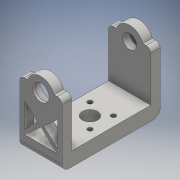
# Autodesk Inventor part: ServoArm
Saved by Autodesk Inventor 2016 (Build 200138000, 138)
## iProperties
Created: 2016-11-10
Part Number: ServoArm
Material: 一般
Document SubType Name: Modeling
Designer: Daisuke
Density: 1 g/cm^3
Appearance: 既定
Author: Daisuke
Autodesk Inventor part; units mm, degrees
ref_plane "YZ Plane" through (0, 0, 0) normal (1, 0, 0) x (0, 1, 0)
ref_plane "XZ Plane" through (0, 0, 0) normal (0, 1, 0) x (-1, 0, 0)
ref_plane "XY Plane" through (0, 0, 0) normal (0, 0, 1) x (1, 0, 0)
sketch "スケッチ1" plane through (0, 0, 0) normal (0, 0, 1) x (1, 0, 0)
  line L0 (-9, 20.9) -> (9, 20.9)
  line L1 (9, 20.9) -> (9, -20.9)
  line L2 (9, -20.9) -> (-9, -20.9)
  line L3 (-9, -20.9) -> (-9, 20.9)
  line L4 (-9, 20.9) -> (9, -20.9) construction
  line L5 (9, 20.9) -> (-9, -20.9) construction
  circle A0 centre (0, 0) radius 3.25
  line L6 (-5, 5) -> (5, 5) construction
  line L7 (5, 5) -> (5, -5) construction
  line L8 (5, -5) -> (-5, -5) construction
  line L9 (-5, -5) -> (-5, 5) construction
  line L10 (-5, 5) -> (5, -5) construction
  line L11 (5, 5) -> (-5, -5) construction
  circle A1 centre (5, 5) radius 1
  circle A2 centre (-5, 5) radius 1
  circle A3 centre (-5, -5) radius 1
  circle A4 centre (5, -5) radius 1
  dimension "d0" = 18
  dimension "d1" = 41.8
  dimension "d2" = 6.5
  dimension "d3" = 10
  dimension "d4" = 10
  dimension "d5" = 2
  dimension "d6" = 2
  dimension "d7" = 2
  dimension "d8" = 2
  constraints: 24 end point, 5 centre point, 5 coincident, 4 midpoint, 4 parallel, 2 horizontal, 2 perpendicular
  measures "d0" distance of L1.end L2.end
  measures "d1" distance of L0.end L1.end
  measures "d2" diameter of A0
  measures "d3" distance of L7.end L8.end
  measures "d4" distance of L6.end L7.end
  measures "d5" diameter of A1
  measures "d6" diameter of A2
  measures "d7" diameter of A3
  measures "d8" diameter of A4
extrude "押し出し1" add sketch "スケッチ1" along normal blind 6
sketch "スケッチ2" plane through (0, 0, 6) normal (0, 0, 1) x (1, 0, 0)
  line L0 (-9, 20.9) -> (9, 20.9)
  line L1 (-9, 9) -> (-9, 20.9)
  line L2 (9, 20.9) -> (-9, 20.9)
  line L3 (-9, 20.9) -> (-9, 16.9)
  line L4 (-9, 16.9) -> (9, 16.9)
  line L5 (9, 16.9) -> (9, 20.9)
  line L6 (9, -9) -> (9, -20.9)
  line L7 (-9, -20.9) -> (-9, -9)
  line L8 (9, -20.9) -> (-9, -20.9)
  line L9 (-9, -20.9) -> (-9, -16.9)
  line L10 (-9, -16.9) -> (9, -16.9)
  line L11 (9, -16.9) -> (9, -20.9)
  point P0 (0, 0)
  point P1 (0, 0)
  dimension "d11" = 4
  dimension "d12" = 4
  constraints: 24 end point, 4 parallel, 2 horizontal, 2 perpendicular, 2 point on line
  measures "d11" distance of L3.end L2.end
  measures "d12" distance of L8.end L9.end
extrude "押し出し2" add sketch "スケッチ2" along normal blind 25
sketch "スケッチ3" plane through (-9, 20.9, 0) normal (0, 1, 0) x (1, 0, 0)
  line L0 (18, -31) -> (18, 0)
  line L1 (0, 0) -> (18, 0)
  line L2 (18, 0) -> (0, 0)
  line L3 (18, -31) -> (18, -25) construction
  line L4 (18, -25) -> (18, -31)
  line L5 (9, -25) -> (15, -25) construction
  line L6 (9, -25) -> (18, -25) construction
  line L7 (16, -27) -> (18, -27)
  line L8 (14.6569, -27) -> (16, -27)
  line L9 (9, -25) -> (9, -31) construction
  line L10 (2, -27) -> (3.3431, -27)
  line L11 (9, -25) -> (0, -25) construction
  line L12 (0, -25) -> (0, -31) construction
  line L13 (0, -25) -> (0, -31)
  circle A0 centre (9, -25) radius 6
  line L14 (18, -6) -> (18, -31)
  line L15 (0, -6) -> (0, -31) construction
  line L16 (18, 0) -> (18, -31) construction
  line L17 (9, 0) -> (9, -25) construction
  line L18 (0, 0) -> (0, -31)
  line L19 (0, -6) -> (0, -31) construction
  line L20 (18, -31) -> (0, -31) construction
  line L21 (0, -31) -> (18, -31) construction
  line L22 (0, -31) -> (18, -31)
  line L23 (18, -31) -> (0, -31) construction
  line L24 (0, -31) -> (18, -31) construction
  line L25 (0, -25) -> (2, -25) construction
  line L26 (2, -25) -> (0, -25) construction
  line L27 (18, -25) -> (16, -25) construction
  line L28 (2, -27) -> (0, -27)
  line L29 (18, -31) -> (18, 0)
  line L30 (0, 0) -> (18, 0)
  line L31 (18, 0) -> (0, 0)
  line L32 (18, -31) -> (18, -25) construction
  line L33 (18, -25) -> (18, -31)
  line L34 (9, -25) -> (15, -25) construction
  line L35 (9, -25) -> (18, -25) construction
  line L36 (16, -27) -> (18, -27)
  line L37 (14.6569, -27) -> (16, -27)
  line L38 (9, -25) -> (9, -31) construction
  line L39 (2, -27) -> (3.3431, -27)
  line L40 (9, -25) -> (0, -25) construction
  line L41 (0, -25) -> (0, -31) construction
  line L42 (0, -25) -> (0, -31)
  circle A1 centre (9, -25) radius 6
  line L43 (18, -6) -> (18, -31)
  line L44 (0, -6) -> (0, -31) construction
  line L45 (18, 0) -> (18, -31) construction
  line L46 (9, 0) -> (9, -25) construction
  line L47 (0, 0) -> (0, -31)
  line L48 (0, -6) -> (0, -31) construction
  line L49 (18, -31) -> (0, -31) construction
  line L50 (0, -31) -> (18, -31) construction
  line L51 (0, -31) -> (18, -31)
  line L52 (18, -31) -> (0, -31) construction
  line L53 (0, -31) -> (18, -31) construction
  line L54 (0, -25) -> (2, -25) construction
  line L55 (2, -25) -> (0, -25) construction
  line L56 (18, -25) -> (16, -25) construction
  line L57 (2, -27) -> (0, -27)
  point P0 (9, -6)
  point P1 (9, -6)
  constraints: 116 end point, 14 point on line, 6 coincident, 4 point on circle, 2 centre point, 2 collinear
extrude "押し出し3" cut sketch "スケッチ3" against normal blind 42 contours L22 A0 L8 L7 L0 | L22 L13 L28 L10 A0
sketch "スケッチ4" plane through (-9, 16.9, 6) normal (0, -1, 0) x (1, 0, 0)
  line L0 (0, 25.0086) -> (0, 19.0086)
  line L1 (0, 25.0086) -> (0, 19.0086) construction
  line L2 (0, 19.0086) -> (0, 25.0086)
  line L3 (9, 19.0086) -> (3, 19.0086) construction
  line L4 (9, 19.0086) -> (0, 19.0086) construction
  line L5 (2, 21.0086) -> (0, 21.0086)
  line L6 (3.3431, 21.0086) -> (2, 21.0086)
  line L7 (9, 19.0086) -> (9, 25.0086) construction
  line L8 (16, 21.0086) -> (14.6569, 21.0086)
  line L9 (9, 19.0086) -> (18, 19.0086) construction
  line L10 (18, 19.0086) -> (18, 25.0086) construction
  line L11 (18, 19.0086) -> (18, 25.0086)
  circle A0 centre (9, 19.0086) radius 6
  line L12 (0, 19.0086) -> (0, 25.0086)
  line L13 (18, 19.0086) -> (18, 25.0086) construction
  line L14 (0, 19.0086) -> (0, 25.0086) construction
  line L15 (9, 0) -> (9, 25) construction
  line L16 (18, 19.0086) -> (18, 25.0086)
  line L17 (18, 0.0086) -> (18, 25.0086) construction
  line L18 (0, 25.0086) -> (18, 25.0086) construction
  line L19 (18, 25.0086) -> (0, 25.0086) construction
  line L20 (18, 25.0086) -> (0, 25.0086)
  line L21 (0, 25.0086) -> (18, 25.0086) construction
  line L22 (18, 25.0086) -> (0, 25.0086) construction
  line L23 (18, 19.0086) -> (16, 19.0086) construction
  line L24 (16, 19.0086) -> (18, 19.0086) construction
  line L25 (0, 19.0086) -> (2, 19.0086) construction
  line L26 (16, 21.0086) -> (18, 21.0086)
  circle A1 centre (9, 19.0086) radius 1.5
  circle A2 centre (9, 19.0086) radius 3
  point P0 (9, -6)
  point P1 (9, 0.0086)
  dimension "d17" = 3
  dimension "d18" = 6
  constraints: 54 end point, 6 point on line, 5 coincident, 3 centre point, 2 point on circle
  measures "d17" diameter of A1
  measures "d18" diameter of A2
extrude "押し出し4" cut sketch "スケッチ4" against normal blind 3 contours A2
sketch "スケッチ5" plane through (-9, 16.9, 6) normal (0, -1, 0) x (1, 0, 0)
  line L0 (0, 25.0086) -> (0, 19.0086)
  line L1 (0, 25.0086) -> (0, 19.0086) construction
  line L2 (0, 19.0086) -> (0, 25.0086)
  line L3 (9, 19.0086) -> (3, 19.0086) construction
  line L4 (9, 19.0086) -> (0, 19.0086) construction
  line L5 (2, 21.0086) -> (0, 21.0086)
  line L6 (3.3431, 21.0086) -> (2, 21.0086)
  line L7 (9, 19.0086) -> (9, 25.0086) construction
  line L8 (16, 21.0086) -> (14.6569, 21.0086)
  line L9 (9, 19.0086) -> (18, 19.0086) construction
  line L10 (18, 19.0086) -> (18, 25.0086) construction
  line L11 (18, 19.0086) -> (18, 25.0086)
  circle A0 centre (9, 19.0086) radius 6
  line L12 (0, 19.0086) -> (0, 25.0086)
  line L13 (18, 19.0086) -> (18, 25.0086) construction
  line L14 (0, 19.0086) -> (0, 25.0086) construction
  line L15 (9, 0) -> (9, 25) construction
  line L16 (18, 19.0086) -> (18, 25.0086)
  line L17 (18, 0.0086) -> (18, 25.0086) construction
  line L18 (0, 25.0086) -> (18, 25.0086) construction
  line L19 (18, 25.0086) -> (0, 25.0086) construction
  line L20 (18, 25.0086) -> (0, 25.0086)
  line L21 (0, 25.0086) -> (18, 25.0086) construction
  line L22 (18, 25.0086) -> (0, 25.0086) construction
  line L23 (18, 19.0086) -> (16, 19.0086) construction
  line L24 (16, 19.0086) -> (18, 19.0086) construction
  line L25 (0, 19.0086) -> (2, 19.0086) construction
  line L26 (16, 21.0086) -> (18, 21.0086)
  circle A1 centre (9, 19.0086) radius 1.5
  circle A2 centre (9, 19.0086) radius 3
  point P0 (9, -6)
  point P1 (9, -6)
  point P2 (9, 0.0086)
  dimension "d21" = 3
  dimension "d22" = 6
  constraints: 54 end point, 6 point on line, 5 coincident, 3 centre point, 2 point on circle
  measures "d21" diameter of A1
  measures "d22" diameter of A2
extrude "押し出し5" cut sketch "スケッチ5" against normal blind 4 contours A1
sketch "スケッチ6" plane through (-9, -16.9, 6) normal (0, 1, 0) x (1, 0, 0)
  line L0 (18, -25.0086) -> (18, -19.0086)
  line L1 (18, -25.0086) -> (18, -19.0086) construction
  line L2 (18, -19.0086) -> (18, -25.0086)
  line L3 (9, -19.0086) -> (15, -19.0086) construction
  line L4 (9, -19.0086) -> (18, -19.0086) construction
  line L5 (16, -21.0086) -> (18, -21.0086)
  line L6 (14.6569, -21.0086) -> (16, -21.0086)
  line L7 (9, -19.0086) -> (9, -25.0086) construction
  line L8 (2, -21.0086) -> (3.3431, -21.0086)
  line L9 (9, -19.0086) -> (0, -19.0086) construction
  line L10 (0, -19.0086) -> (0, -25.0086) construction
  line L11 (0, -19.0086) -> (0, -25.0086)
  circle A0 centre (9, -19.0086) radius 6
  line L12 (18, -19.0086) -> (18, -25.0086)
  line L13 (0, -19.0086) -> (0, -25.0086) construction
  line L14 (18, -19.0086) -> (18, -25.0086) construction
  line L15 (9, 0) -> (9, -25) construction
  line L16 (0, -19.0086) -> (0, -25.0086)
  line L17 (0, -0.0086) -> (0, -25.0086) construction
  line L18 (18, -25.0086) -> (0, -25.0086) construction
  line L19 (0, -25.0086) -> (18, -25.0086) construction
  line L20 (0, -25.0086) -> (18, -25.0086)
  line L21 (18, -25.0086) -> (0, -25.0086) construction
  line L22 (0, -25.0086) -> (18, -25.0086) construction
  line L23 (0, -19.0086) -> (2, -19.0086) construction
  line L24 (2, -19.0086) -> (0, -19.0086) construction
  line L25 (18, -19.0086) -> (16, -19.0086) construction
  line L26 (2, -21.0086) -> (0, -21.0086)
  circle A1 centre (9, -19.0086) radius 3.5
  circle A2 centre (9, -19.0086) radius 4.5
  line L27 (18, -25.0086) -> (18, -19.0086)
  line L28 (18, -25.0086) -> (18, -19.0086) construction
  line L29 (18, -19.0086) -> (18, -25.0086)
  line L30 (9, -19.0086) -> (15, -19.0086) construction
  line L31 (9, -19.0086) -> (18, -19.0086) construction
  line L32 (16, -21.0086) -> (18, -21.0086)
  line L33 (14.6569, -21.0086) -> (16, -21.0086)
  line L34 (9, -19.0086) -> (9, -25.0086) construction
  line L35 (2, -21.0086) -> (3.3431, -21.0086)
  line L36 (9, -19.0086) -> (0, -19.0086) construction
  line L37 (0, -19.0086) -> (0, -25.0086) construction
  line L38 (0, -19.0086) -> (0, -25.0086)
  circle A3 centre (9, -19.0086) radius 6
  line L39 (18, -19.0086) -> (18, -25.0086)
  line L40 (0, -19.0086) -> (0, -25.0086) construction
  line L41 (18, -19.0086) -> (18, -25.0086) construction
  line L42 (9, 0) -> (9, -25) construction
  line L43 (0, -19.0086) -> (0, -25.0086)
  line L44 (0, -0.0086) -> (0, -25.0086) construction
  line L45 (18, -25.0086) -> (0, -25.0086) construction
  line L46 (0, -25.0086) -> (18, -25.0086) construction
  line L47 (0, -25.0086) -> (18, -25.0086)
  line L48 (18, -25.0086) -> (0, -25.0086) construction
  line L49 (0, -25.0086) -> (18, -25.0086) construction
  line L50 (0, -19.0086) -> (2, -19.0086) construction
  line L51 (2, -19.0086) -> (0, -19.0086) construction
  line L52 (18, -19.0086) -> (16, -19.0086) construction
  line L53 (2, -21.0086) -> (0, -21.0086)
  circle A4 centre (9, -19.0086) radius 3.5
  circle A5 centre (9, -19.0086) radius 4.5
  point P0 (9, 6)
  point P1 (9, -0.0086)
  point P2 (9, -0.0086)
  dimension "d25" = 7
  dimension "d26" = 9
  dimension "d27" = 7
  dimension "d28" = 9
  constraints: 108 end point, 12 point on line, 10 coincident, 6 centre point, 4 point on circle
  measures "d25" diameter of A1
  measures "d26" diameter of A2
  measures "d27" diameter of A4
  measures "d28" diameter of A5
extrude "押し出し6" cut sketch "スケッチ6" against normal blind 3 contours A2
sketch "スケッチ7" plane through (-9, -16.9, 6) normal (0, 1, 0) x (1, 0, 0)
  line L0 (18, -25.0086) -> (18, -19.0086)
  line L1 (18, -25.0086) -> (18, -19.0086) construction
  line L2 (18, -19.0086) -> (18, -25.0086)
  line L3 (9, -19.0086) -> (15, -19.0086) construction
  line L4 (9, -19.0086) -> (18, -19.0086) construction
  line L5 (16, -21.0086) -> (18, -21.0086)
  line L6 (14.6569, -21.0086) -> (16, -21.0086)
  line L7 (9, -19.0086) -> (9, -25.0086) construction
  line L8 (2, -21.0086) -> (3.3431, -21.0086)
  line L9 (9, -19.0086) -> (0, -19.0086) construction
  line L10 (0, -19.0086) -> (0, -25.0086) construction
  line L11 (0, -19.0086) -> (0, -25.0086)
  circle A0 centre (9, -19.0086) radius 6
  line L12 (18, -19.0086) -> (18, -25.0086)
  line L13 (0, -19.0086) -> (0, -25.0086) construction
  line L14 (18, -19.0086) -> (18, -25.0086) construction
  line L15 (9, 0) -> (9, -25) construction
  line L16 (0, -19.0086) -> (0, -25.0086)
  line L17 (0, -0.0086) -> (0, -25.0086) construction
  line L18 (18, -25.0086) -> (0, -25.0086) construction
  line L19 (0, -25.0086) -> (18, -25.0086) construction
  line L20 (0, -25.0086) -> (18, -25.0086)
  line L21 (18, -25.0086) -> (0, -25.0086) construction
  line L22 (0, -25.0086) -> (18, -25.0086) construction
  line L23 (0, -19.0086) -> (2, -19.0086) construction
  line L24 (2, -19.0086) -> (0, -19.0086) construction
  line L25 (18, -19.0086) -> (16, -19.0086) construction
  line L26 (2, -21.0086) -> (0, -21.0086)
  circle A1 centre (9, -19.0086) radius 3.5
  circle A2 centre (9, -19.0086) radius 4.5
  line L27 (18, -25.0086) -> (18, -19.0086)
  line L28 (18, -25.0086) -> (18, -19.0086) construction
  line L29 (18, -19.0086) -> (18, -25.0086)
  line L30 (9, -19.0086) -> (15, -19.0086) construction
  line L31 (9, -19.0086) -> (18, -19.0086) construction
  line L32 (16, -21.0086) -> (18, -21.0086)
  line L33 (14.6569, -21.0086) -> (16, -21.0086)
  line L34 (9, -19.0086) -> (9, -25.0086) construction
  line L35 (2, -21.0086) -> (3.3431, -21.0086)
  line L36 (9, -19.0086) -> (0, -19.0086) construction
  line L37 (0, -19.0086) -> (0, -25.0086) construction
  line L38 (0, -19.0086) -> (0, -25.0086)
  circle A3 centre (9, -19.0086) radius 6
  line L39 (18, -19.0086) -> (18, -25.0086)
  line L40 (0, -19.0086) -> (0, -25.0086) construction
  line L41 (18, -19.0086) -> (18, -25.0086) construction
  line L42 (9, 0) -> (9, -25) construction
  line L43 (0, -19.0086) -> (0, -25.0086)
  line L44 (0, -0.0086) -> (0, -25.0086) construction
  line L45 (18, -25.0086) -> (0, -25.0086) construction
  line L46 (0, -25.0086) -> (18, -25.0086) construction
  line L47 (0, -25.0086) -> (18, -25.0086)
  line L48 (18, -25.0086) -> (0, -25.0086) construction
  line L49 (0, -25.0086) -> (18, -25.0086) construction
  line L50 (0, -19.0086) -> (2, -19.0086) construction
  line L51 (2, -19.0086) -> (0, -19.0086) construction
  line L52 (18, -19.0086) -> (16, -19.0086) construction
  line L53 (2, -21.0086) -> (0, -21.0086)
  circle A4 centre (9, -19.0086) radius 3.5
  circle A5 centre (9, -19.0086) radius 4.5
  point P0 (9, 6)
  point P1 (9, 6)
  point P2 (9, -0.0086)
  point P3 (9, -0.0086)
  dimension "d31" = 7
  dimension "d32" = 9
  dimension "d33" = 7
  dimension "d34" = 9
  constraints: 108 end point, 12 point on line, 10 coincident, 6 centre point, 4 point on circle
  measures "d31" diameter of A1
  measures "d32" diameter of A2
  measures "d33" diameter of A4
  measures "d34" diameter of A5
extrude "押し出し7" cut sketch "スケッチ7" against normal blind 4 contours A1
sketch "スケッチ8" plane through (-9, -16.9, 6) normal (0, 1, 0) x (1, 0, 0)
  line L0 (18, -25.0086) -> (18, -19.0086)
  line L1 (18, -25.0086) -> (18, -19.0086) construction
  line L2 (18, -19.0086) -> (18, -25.0086)
  line L3 (9, -19.0086) -> (15, -19.0086) construction
  line L4 (9, -19.0086) -> (18, -19.0086) construction
  line L5 (16, -21.0086) -> (18, -21.0086)
  line L6 (14.6569, -21.0086) -> (16, -21.0086)
  line L7 (9, -19.0086) -> (9, -25.0086) construction
  line L8 (2, -21.0086) -> (3.3431, -21.0086)
  line L9 (9, -19.0086) -> (0, -19.0086) construction
  line L10 (0, -19.0086) -> (0, -25.0086) construction
  line L11 (0, -19.0086) -> (0, -25.0086)
  circle A0 centre (9, -19.0086) radius 6
  line L12 (18, -19.0086) -> (18, -25.0086)
  line L13 (0, -19.0086) -> (0, -25.0086) construction
  line L14 (18, -19.0086) -> (18, -25.0086) construction
  line L15 (9, 0) -> (9, -25) construction
  line L16 (0, -19.0086) -> (0, -25.0086)
  line L17 (0, -0.0086) -> (0, -25.0086) construction
  line L18 (18, -25.0086) -> (0, -25.0086) construction
  line L19 (0, -25.0086) -> (18, -25.0086) construction
  line L20 (0, -25.0086) -> (18, -25.0086)
  line L21 (18, -25.0086) -> (0, -25.0086) construction
  line L22 (0, -25.0086) -> (18, -25.0086) construction
  line L23 (0, -19.0086) -> (2, -19.0086) construction
  line L24 (2, -19.0086) -> (0, -19.0086) construction
  line L25 (18, -19.0086) -> (16, -19.0086) construction
  line L26 (2, -21.0086) -> (0, -21.0086)
  circle A1 centre (9, -19.0086) radius 3.5
  circle A2 centre (9, -19.0086) radius 4.5
  line L27 (18, -19.0086) -> (16, -19.0086) construction
  line L28 (0, 0) -> (18, 0) construction
  line L29 (18, 0) -> (18, -21) construction
  line L30 (0, 0) -> (18, 0) construction
  line L31 (18, 0) -> (18, -14.5086) construction
  line L32 (0, -14.5086) -> (0, 0) construction
  line L33 (18, 0) -> (16, 0) construction
  line L34 (0, 0) -> (2, 0) construction
  line L35 (16, 0) -> (2, 0)
  line L36 (2, -2) -> (2, -12.5086)
  line L37 (16, -12.5086) -> (16, -2)
  line L38 (16, -12.5086) -> (10.1192, -7.2543)
  line L39 (9, -6.2543) -> (2, 0)
  line L40 (16, -2) -> (10.1192, -7.2543)
  line L41 (9, -8.2543) -> (2, -14.5086)
  line L42 (2, -12.5086) -> (7.8808, -7.2543)
  line L43 (9, -6.2543) -> (16, 0)
  line L44 (2, -2) -> (7.8808, -7.2543)
  line L45 (9, -8.2543) -> (16, -14.5086)
  line L46 (2, -14.5086) -> (9, -14.5086)
  line L47 (12.9686, -14.5086) -> (16, -14.5086)
  line L48 (18, -14.5086) -> (9, -14.5086) construction
  line L49 (5.0314, -14.5086) -> (0, -14.5086) construction
  point P0 (9, 6)
  point P1 (9, -0.0086)
  dimension "d38" = 9
  dimension "d37" = 7
  dimension "d39" = 2
  dimension "d40" = 2
  constraints: 100 end point, 14 parallel, 12 point on line, 5 coincident, 4 point on circle, 2 centre point, 2 horizontal, 2 perpendicular, 1 collinear, 1 vertical alignment, 2 other
  measures "d37" diameter of A1
  measures "d39" distance of L0.end L25.end
  measures "d40" distance of L28.start L34.end
extrude "押し出し8" cut sketch "スケッチ8" against normal blind 4 contours L43 L39 L35 | L44 L42 L36 | L38 L40 L37
fillet "フィレット1" radius 2 4 edges at (-9, 18.9, 27) (-9, -18.9, 27) (9, -18.9, 27) (9, 18.9, 27)
fillet "フィレット2" radius 3 2 edges at (0, -20.9, 0) (0, 20.9, 0)
